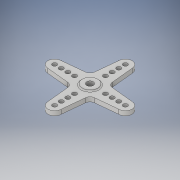
# Autodesk Inventor part: palonnierServo
Saved by Autodesk Inventor 2019 (Build 230136000, 136)
## iProperties
Created: 2021-01-22
Part Number: palonnierServo
Material: Générique
Document SubType Name: Modeling
Designer: tom.mousset
Density: 1 g/cm^3
Appearance: Par défaut
Author: tom.mousset
Autodesk Inventor part; units mm, degrees
ref_plane "YZ Plane" through (0, 0, 0) normal (1, 0, 0) x (0, 1, 0)
ref_plane "XZ Plane" through (0, 0, 0) normal (0, 1, 0) x (-1, 0, 0)
ref_plane "XY Plane" through (0, 0, 0) normal (0, 0, 1) x (1, 0, 0)
sketch "Esquisse1" plane through (0, 0, 0) normal (0, 1, 0) x (-1, 0, 0)
  circle A0 centre (0, 0) radius 19 construction
  circle A1 centre (0, 0) radius 6.75 construction
  line L0 (0, 0) -> (0, -19) construction
  line L1 (0, 0) -> (-13.435, -13.435) construction
  line L2 (0, 0) -> (19, 0) construction
  circle A2 centre (0, -7) radius 1 construction
  circle A3 centre (0, -10) radius 1 construction
  circle A4 centre (0, -13) radius 1 construction
  circle A5 centre (0, -16) radius 1 construction
  circle A6 centre (0, -16) radius 3 construction
  arc A7 (-3, -16) -> (0, -19) centre (0, -16) ccw
  line L3 (-9.6742, -0.3258) -> (-4, -6) construction
  line L4 (-4, -6) -> (-5, -5) construction
  line L5 (-5, -5) -> (-6, -4) construction
  arc A8 (-4, -6) -> (-6, -4) centre (-6.2222, -6.2222) ccw construction
  arc A9 (-4, -6) -> (-4.643, -4.643) centre (-6.2222, -6.2222) ccw
  arc A10 (0, -15) -> (0, -17) centre (0, -16) ccw
  arc A11 (0, -12) -> (0, -14) centre (0, -13) ccw
  arc A12 (0, -9) -> (0, -11) centre (0, -10) ccw
  arc A13 (0, -6) -> (0, -8) centre (0, -7) ccw
  line L6 (0, 0) -> (0, -6)
  line L7 (0, -8) -> (0, -9)
  line L8 (0, -11) -> (0, -12)
  line L9 (0, -14) -> (0, -15)
  line L10 (0, -17) -> (0, -19)
  line L11 (-4.643, -4.643) -> (0, 0)
  line L12 (-3, -16) -> (-4, -6)
  dimension "d0" = 38
  dimension "d1" = 13.5
  dimension "d2" = 135
  dimension "d3" = 2
  dimension "d4" = 7
  dimension "d5" = 2
  dimension "d6" = 10
  dimension "d7" = 2
  dimension "d8" = 13
  dimension "d9" = 2
  dimension "d10" = 16
  dimension "d11" = 4
  dimension "d12" = 13
  constraints: 25 point on circle, 24 end point, 13 centre point, 11 coincident, 4 point on line, 4 vertical, 2 collinear, 2 equal length, 1 horizontal, 1 horizontal alignment, 1 vertical alignment, 18 other
  measures "d0" diameter of A0
  measures "d1" diameter of A1
  measures "d2" angle of L1 L2
  measures "d3" diameter of A2
  measures "d4" distance of point (0, 0) A2.centre
  measures "d5" diameter of A3
  measures "d6" distance of point (0, 0) A3.centre
  measures "d7" diameter of A4
  measures "d8" distance of point (0, 0) A4.centre
  measures "d9" diameter of A5
  measures "d10" distance of point (0, 0) A5.centre
  measures "d11" horizontal distance of point (0, 0) A8.start
  measures "d12" vertical distance of A0.start A8.start
extrude "Extrusion1" add sketch "Esquisse1" along normal blind 2
mirror "Symétrie1" about plane through (0, 0, 0) normal (1, 0, 0) of "Extrusion1"
pattern_circular "Réseau circulaire1" count 4 over 360 about axis through (0, -10, 0) along (0, 1, 0) of "Extrusion1", "Symétrie1"
sketch "Esquisse2" plane through (0, 0, 0) normal (0, -1, 0) x (1, 0, 0)
  circle A0 centre (0, 0) radius 5
  circle A1 centre (0, 0) radius 2.5
  dimension "d19" = 10
  dimension "d22" = 5
  constraints: 2 centre point, 2 coincident
  measures "d19" diameter of A0
  measures "d22" diameter of A1
extrude "Extrusion2" add sketch "Esquisse2" along normal blind 2.5
fillet "Congé1" radius 2 1 edges at (-5, -2.5, 0) inverted yes
sketch "Esquisse3" plane through (0, 2, 0) normal (0, 1, 0) x (1, 0, 0)
  circle A0 centre (0, 0) radius 3.5
  dimension "d24" = 7
  constraints: 1 centre point, 1 coincident
  measures "d24" diameter of A0
extrude "Extrusion3" add sketch "Esquisse3" along normal blind 0.5
fillet "Congé2" radius 0.5 1 edges at (-3.5, 2, 0)
sketch "Esquisse4" plane through (0, 2.5, 0) normal (0, 1, 0) x (1, 0, 0)
  circle A0 centre (0, 0) radius 1.5
  dimension "d28" = 3
  constraints: 1 centre point, 1 coincident
  measures "d28" diameter of A0
extrude "Extrusion4" cut sketch "Esquisse4" against normal blind 10
